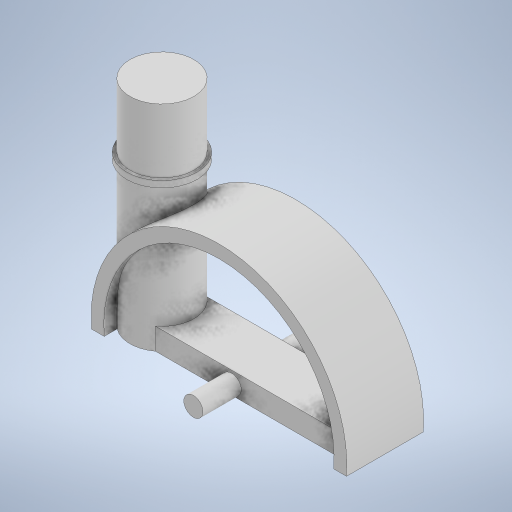
# Autodesk Inventor part: Wheel sheild (H)
Saved by Autodesk Inventor 2023 (Build 270158030, 158C)
## iProperties
Created: 2023-03-03
Part Number: Wheel sheild (H)
Material: Generic
Document SubType Name: Modeling
Designer: mpino
Density: 1 g/cm^3
Appearance: Default
Author: mpino
Autodesk Inventor part; units mm, degrees
ref_plane "YZ Plane" through (0, 0, 0) normal (1, 0, 0) x (0, 1, 0)
ref_plane "XZ Plane" through (0, 0, 0) normal (0, 1, 0) x (-1, 0, 0)
ref_plane "XY Plane" through (0, 0, 0) normal (0, 0, 1) x (1, 0, 0)
sketch "Sketch1" plane through (0, 0, 0) normal (0, 1, 0) x (-1, 0, 0)
  circle A0 centre (0, 0) radius 6.35
  dimension "d0" = 12.7
  constraints: 1 centre point, 1 coincident
  measures "d0" diameter of A0
extrude "Extrusion1" add sketch "Sketch1" along normal blind 12.7
sketch "Sketch2" plane through (0, 0, 0) normal (0, -1, 0) x (1, 0, 0)
  circle A0 centre (0, 0) radius 6.985
  dimension "d3" = 13.97
  constraints: 1 centre point, 1 coincident
  measures "d3" diameter of A0
extrude "Extrusion2" add sketch "Sketch2" along normal blind 1.27
sketch "Sketch3" plane through (0, -1.27, 0) normal (0, -1, 0) x (1, 0, 0)
  circle A0 centre (0, 0) radius 6.35
  dimension "d6" = 12.7
  constraints: 1 centre point, 1 coincident
  measures "d6" diameter of A0
extrude "Extrusion3" add sketch "Sketch3" along normal blind 28.575
sketch "Sketch4" plane through (0, 0, 0) normal (0, 0, 1) x (1, 0, 0)
  line L0 (-6.35, -29.845) -> (6.35, -29.845) projected
  line L1 (-6.35, -29.845) -> (-6.35, -1.27)
  line L2 (-6.985, -1.27) -> (6.985, -1.27) projected
  line L3 (-6.35, -1.27) -> (-6.35, -29.845) projected
  circle A0 centre (18.9357, -27.94) radius 25.4
  circle A1 centre (18.9357, -27.94) radius 22.86
  line L4 (-6.3928, -29.845) -> (44.2642, -29.845)
  point P0 (0, 0)
  point P1 (0, -1.27)
  point P2 (41.7162, -29.845)
  point P3 (-3.8448, -29.845)
  point P4 (-6.35, -25.5331)
  dimension "d11" = 45.72
  dimension "d12" = 26.67
  dimension "d13" = 50.8
  dimension "d14" = 25.2857
  constraints: 4 end point, 3 point on line, 2 centre point, 2 point on circle, 1 coincident, 1 midpoint, 1 vertical
  measures "d11" diameter of A1
  measures "d12" vertical distance of point (0, -1.27) A0.centre
  measures "d13" diameter of A0
  measures "d14" distance from line of L1 A0.centre
extrude "Extrusion4" add sketch "Sketch4" along normal mid plane 15.24 contours L1 A0 L4 A1 L0
sketch "Sketch5" plane through (-6.35, -29.845, 7.62) normal (-1, 0, 0) x (0, 0, 1)
  line L0 (-2.54, 4.318) -> (-2.54, 0)
  line L1 (-2.54, 0) -> (-12.7, 0)
  line L2 (-12.7, 0) -> (-12.7, 4.318)
  line L3 (0, 4.3119) -> (0, 0) projected
  line L4 (-15.24, 0) -> (-15.24, 4.3119) projected
  line L5 (-7.62, 4.3119) -> (0, 4.3119) projected
  line L6 (-12.7, 4.3119) -> (-2.54, 4.3119)
  point P0 (-7.62, 29.845)
  point P1 (-2.5663, 0)
  point P2 (-3.81, 4.3119)
  point P3 (-2.54, 4.3119)
  dimension "d17" = 2.54
  dimension "d18" = 2.54
  dimension "d21" = 4.3119
  dimension "d22" = 0.0061
  dimension "d23" = 0.0061
  constraints: 8 end point, 3 point on line, 1 midpoint, 1 parallel, 1 perpendicular
  measures "d17" distance between parallel lines of L3 L0
  measures "d18" distance between parallel lines of L4 L2
  measures "d21" distance between parallel lines of L5 L1
  measures "d22" distance from line of L0.start L5
  measures "d23" distance from line of L2.end L5
extrude "Extrusion5" add sketch "Sketch5" against normal blind 50.165
sketch "Sketch6" plane through (0, 0, 0) normal (0, 0, 1) x (1, 0, 0)
  arc A0 (41.7162, -29.845) -> (-3.8448, -29.845) centre (18.9357, -27.94) ccw projected
  circle A1 centre (18.9357, -27.94) radius 1.905
  point P0 (0, 0)
  point P1 (4.5348, -10.1863)
  point P2 (0, -15.133)
  dimension "d26" = 3.81
  constraints: 1 centre point, 1 coincident
  measures "d26" diameter of A1
extrude "Extrusion6" add sketch "Sketch6" along normal mid plane 25.4
body "Solid1"
